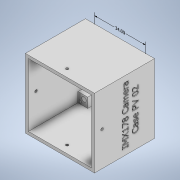
# Autodesk Inventor part: IMX178 Camera Case Base
Saved by Autodesk Inventor 2022.1 (Build 261234000, 234)
## iProperties
Created: 2021-07-23
Part Number: IMX178 Camera Case Base
Material: Generic
Document SubType Name: Modeling
Designer: robst
Density: 1 g/cm^3
Appearance: Default
Author: robst
Autodesk Inventor part; units mm, degrees
ref_plane "YZ Plane" through (0, 0, 0) normal (1, 0, 0) x (0, 1, 0)
ref_plane "XZ Plane" through (0, 0, 0) normal (0, 1, 0) x (-1, 0, 0)
ref_plane "XY Plane" through (0, 0, 0) normal (0, 0, 1) x (1, 0, 0)
sketch "Sketch8" plane through (0, 0, 0) normal (0, 0, 1) x (1, 0, 0)
  line L0 (-17, -17) -> (17, -17) construction
  line L1 (17, -17) -> (17, 17) construction
  line L2 (17, 17) -> (-17, 17) construction
  line L3 (-17, 17) -> (-17, -17) construction
  line L4 (-17, -17) -> (17, 17) construction
  line L5 (17, -17) -> (-17, 17) construction
  circle A0 centre (-17, 17) radius 1.5
  circle A1 centre (17, 17) radius 1.5
  circle A2 centre (17, -17) radius 1.5
  circle A3 centre (-17, -17) radius 1.5
  line L6 (-21, -21) -> (21, -21)
  line L7 (21, -21) -> (21, 21)
  line L8 (21, 21) -> (-21, 21)
  line L9 (-21, 21) -> (-21, -21)
  line L10 (-21, -21) -> (21, 21) construction
  line L11 (21, -21) -> (-21, 21) construction
  line L12 (-23, -23) -> (23, -23)
  line L13 (23, -23) -> (23, 23)
  line L14 (23, 23) -> (-23, 23)
  line L15 (-23, 23) -> (-23, -23)
  line L16 (-23, -23) -> (23, 23) construction
  line L17 (23, -23) -> (-23, 23) construction
  line L18 (0, 0) -> (9.8286, 0)
  line L19 (-14.5, -14.5) -> (14.5, -14.5) construction
  line L20 (14.5, -14.5) -> (14.5, 14.5) construction
  line L21 (14.5, 14.5) -> (-14.5, 14.5) construction
  line L22 (-14.5, 14.5) -> (-14.5, -14.5) construction
  line L23 (-14.5, -14.5) -> (14.5, 14.5) construction
  line L24 (14.5, -14.5) -> (-14.5, 14.5) construction
  line L25 (-21, 21) -> (-14.5, 21)
  line L26 (-14.5, 21) -> (-14.5, 14.5)
  line L27 (-14.5, 14.5) -> (-21, 14.5)
  line L28 (-21, 14.5) -> (-21, 21)
  line L29 (21, 21) -> (14.5, 21)
  line L30 (14.5, 21) -> (14.5, 14.5)
  line L31 (14.5, 14.5) -> (21, 14.5)
  line L32 (21, 14.5) -> (21, 21)
  line L33 (21, -21) -> (14.5, -21)
  line L34 (14.5, -21) -> (14.5, -14.5)
  line L35 (14.5, -14.5) -> (21, -14.5)
  line L36 (21, -14.5) -> (21, -21)
  line L37 (-21, -21) -> (-14.5, -21)
  line L38 (-14.5, -21) -> (-14.5, -14.5)
  line L39 (-14.5, -14.5) -> (-21, -14.5)
  line L40 (-21, -14.5) -> (-21, -21)
  point P0 (-23, 0)
  dimension "d46" = 34
  dimension "d47" = 34
  dimension "d48" = 3
  dimension "d49" = 42
  dimension "d50" = 42
  dimension "d51" = 2
  dimension "d52" = 2
  dimension "d53" = 29
  dimension "d54" = 29
  constraints: 82 end point, 16 parallel, 9 midpoint, 8 horizontal, 8 perpendicular, 4 centre point, 4 coincident, 3 equal radius, 2 point on line
  measures "d46" distance of L0.start L0.end
  measures "d47" distance of L2.end L0.start
  measures "d48" diameter of A0
  measures "d49" distance of L7.end L8.end
  measures "d50" distance of L6.end L7.end
  measures "d51" distance between parallel lines of L8 L14
  measures "d52" distance from line of point (-23, 0) L9
  measures "d53" distance of L19.start L19.end
  measures "d54" distance of L20.end L19.end
extrude "Extrusion9" add sketch "Sketch8" against normal blind 15 contours L9 L39 L38 L6 | L34 L35 L7 L6 | L9 L8 L26 L27 | L31 L30 L8 L7 | L15 L14 L13 L12
sketch "Sketch9" plane through (0, 0, 0) normal (0, 0, 1) x (1, 0, 0)
  line L0 (21, 14.5) -> (21, -14.5) projected
  line L1 (-14.5, 21) -> (14.5, 21) projected
  line L2 (-21, -14.5) -> (-21, 14.5) projected
  line L3 (14.5, -21) -> (-14.5, -21) projected
  line L4 (-23, -23) -> (23, -23) projected
  line L5 (23, -23) -> (23, 23) projected
  line L6 (23, 23) -> (-23, 23) projected
  line L7 (-23, 23) -> (-23, -23) projected
  line L8 (-21, -21) -> (21, -21)
  line L9 (21, -21) -> (21, 21)
  line L10 (21, 21) -> (-21, 21)
  line L11 (-21, 21) -> (-21, -21)
  line L12 (-21, -21) -> (21, 21) construction
  line L13 (21, -21) -> (-21, 21) construction
  line L14 (-23, -23) -> (23, -23)
  line L15 (23, -23) -> (23, 23)
  line L16 (23, 23) -> (-23, 23)
  line L17 (-23, 23) -> (-23, -23)
  line L18 (-23, -23) -> (23, 23) construction
  line L19 (23, -23) -> (-23, 23) construction
  point P0 (0, 0)
  constraints: 24 end point, 4 midpoint, 4 parallel, 2 perpendicular
extrude "Extrusion10" add sketch "Sketch9" along normal blind 25
sketch "Sketch10" plane through (23, -23, -15) normal (1, 0, 0) x (0, 0, -1)
  line L0 (-40, 0) -> (0, 0) construction
  line L1 (-20, 0) -> (-20, 46) construction
  line L2 (0, 46) -> (-40, 46) construction
  line L3 (-17.5, 5.4068) -> (-17.5, 3.8574)
  line L4 (-17.5, 3.8574) -> (-17.9084, 3.8574)
  line L5 (-17.9084, 3.8574) -> (-17.9084, 4.3663)
  line L6 (-17.9084, 4.3663) -> (-21.0916, 4.3663)
  line L7 (-21.0916, 4.3663) -> (-21.0916, 3.8574)
  line L8 (-21.0916, 3.8574) -> (-21.5, 3.8574)
  line L9 (-21.5, 3.8574) -> (-21.5, 5.4068)
  line L10 (-21.5, 5.4068) -> (-21.0916, 5.4068)
  line L11 (-21.0916, 5.4068) -> (-21.0916, 4.8979)
  line L12 (-21.0916, 4.8979) -> (-17.9084, 4.8979)
  line L13 (-17.9084, 4.8979) -> (-17.9084, 5.4068)
  line L14 (-17.9084, 5.4068) -> (-17.5, 5.4068)
  line L15 (-17.5, 9.4943) -> (-17.5, 8.9627)
  line L16 (-17.5, 8.9627) -> (-20.9457, 8.9627)
  line L17 (-20.9457, 8.9627) -> (-18.6021, 7.919)
  line L18 (-18.6021, 7.919) -> (-18.6021, 7.5948)
  line L19 (-18.6021, 7.5948) -> (-20.9457, 6.5608)
  line L20 (-20.9457, 6.5608) -> (-17.5, 6.5608)
  line L21 (-17.5, 6.5608) -> (-17.5, 6.0648)
  line L22 (-17.5, 6.0648) -> (-21.5, 6.0648)
  line L23 (-21.5, 6.0648) -> (-21.5, 6.7909)
  line L24 (-21.5, 6.7909) -> (-19.2731, 7.7893)
  line L25 (-19.2731, 7.7893) -> (-21.5, 8.7553)
  line L26 (-21.5, 8.7553) -> (-21.5, 9.4943)
  line L27 (-21.5, 9.4943) -> (-17.5, 9.4943)
  line L28 (-17.5, 13.0697) -> (-17.5, 12.4603)
  line L29 (-17.5, 12.4603) -> (-19.0948, 11.4878)
  line L30 (-19.0948, 11.4878) -> (-17.5, 10.4959)
  line L31 (-17.5, 10.4959) -> (-17.5, 9.9222)
  line L32 (-17.5, 9.9222) -> (-19.5032, 11.1961)
  line L33 (-19.5032, 11.1961) -> (-21.5, 9.9611)
  line L34 (-21.5, 9.9611) -> (-21.5, 10.5705)
  line L35 (-21.5, 10.5705) -> (-19.9344, 11.5235)
  line L36 (-19.9344, 11.5235) -> (-21.5, 12.4959)
  line L37 (-21.5, 12.4959) -> (-21.5, 13.0697)
  line L38 (-21.5, 13.0697) -> (-19.5292, 11.8185)
  line L39 (-19.5292, 11.8185) -> (-17.5, 13.0697)
  line L40 (-17.5, 15.6499) -> (-17.5, 13.6985)
  line L41 (-17.5, 13.6985) -> (-17.9084, 13.6985)
  line L42 (-17.9084, 13.6985) -> (-17.9084, 14.4246)
  line L43 (-17.9084, 14.4246) -> (-20.5891, 14.4246)
  line L44 (-20.5891, 14.4246) -> (-20.5891, 13.6985)
  line L45 (-20.5891, 13.6985) -> (-20.9554, 13.6985)
  spline S0 degree 2 poles (-20.9554, 13.6985) (-20.9554, 14.1102) (-21.1888, 14.4992) (-21.513, 14.5251) knots 0 0 0 1 2 2 2
  line L46 (-21.513, 14.5251) -> (-21.513, 14.94)
  line L47 (-21.513, 14.94) -> (-17.9084, 14.94)
  line L48 (-17.9084, 14.94) -> (-17.9084, 15.6499)
  line L49 (-17.9084, 15.6499) -> (-17.5, 15.6499)
  line L50 (-20.9003, 18.8979) -> (-17.5, 17.1669)
  line L51 (-17.5, 17.1669) -> (-17.5, 16.5964)
  line L52 (-17.5, 16.5964) -> (-21.03, 18.4246)
  line L53 (-21.03, 18.4246) -> (-21.03, 16.3598)
  line L54 (-21.03, 16.3598) -> (-21.5, 16.3598)
  line L55 (-21.5, 16.3598) -> (-21.5, 18.8979)
  line L56 (-21.5, 18.8979) -> (-20.9003, 18.8979)
  spline S1 degree 2 poles (-17.4092, 20.5964) (-17.4092, 20.2982) (-17.5875, 19.8088) (-17.7528, 19.637) knots 0 0 0 1 2 2 2
  spline S2 degree 2 poles (-17.7528, 19.637) (-17.9149, 19.4684) (-18.3558, 19.2934) (-18.6053, 19.2934) knots 0 0 0 1 2 2 2
  spline S3 degree 2 poles (-18.6053, 19.2934) (-18.9295, 19.2934) (-19.4741, 19.6402) (-19.6361, 19.9708) knots 0 0 0 1 2 2 2
  line L57 (-19.6361, 19.9708) -> (-19.6524, 19.9708)
  spline S4 degree 2 poles (-19.6524, 19.9708) (-19.8241, 19.6759) (-20.2326, 19.3906) (-20.5373, 19.3906) knots 0 0 0 1 2 2 2
  spline S5 degree 2 poles (-20.5373, 19.3906) (-20.9878, 19.3906) (-21.5908, 20.0713) (-21.5908, 20.5964) knots 0 0 0 1 2 2 2
  spline S6 degree 2 poles (-21.5908, 20.5964) (-21.5908, 21.141) (-21.0203, 21.799) (-20.5729, 21.799) knots 0 0 0 1 2 2 2
  spline S7 degree 2 poles (-20.5729, 21.799) (-20.3039, 21.799) (-19.7788, 21.4846) (-19.6297, 21.1896) knots 0 0 0 1 2 2 2
  line L58 (-19.6297, 21.1896) -> (-19.6135, 21.1896)
  spline S8 degree 2 poles (-19.6135, 21.1896) (-19.4514, 21.5397) (-18.9846, 21.8995) (-18.6151, 21.8995) knots 0 0 0 1 2 2 2
  spline S9 degree 2 poles (-18.6151, 21.8995) (-18.1029, 21.8995) (-17.4092, 21.154) (-17.4092, 20.5964) knots 0 0 0 1 2 2 2
  spline S10 degree 2 poles (-18.5632, 21.3485) (-18.8096, 21.3485) (-19.1013, 21.154) (-19.2504, 20.8784) knots 0 0 0 1 2 2 2
  spline S11 degree 2 poles (-19.2504, 20.8784) (-19.3023, 20.7877) (-19.4222, 20.483) (-19.5, 20.2917) knots 0 0 0 1 2 2 2
  spline S12 degree 2 poles (-19.5, 20.2917) (-19.3541, 20.0713) (-18.9198, 19.8347) (-18.6442, 19.8347) knots 0 0 0 1 2 2 2
  spline S13 degree 2 poles (-18.6442, 19.8347) (-18.2812, 19.8347) (-17.8079, 20.2723) (-17.8079, 20.6029) knots 0 0 0 1 2 2 2
  spline S14 degree 2 poles (-17.8079, 20.6029) (-17.8079, 20.94) (-18.2131, 21.3485) (-18.5632, 21.3485) knots 0 0 0 1 2 2 2
  spline S15 degree 2 poles (-20.5665, 21.2739) (-20.8355, 21.2739) (-21.1953, 20.9141) (-21.1953, 20.5932) knots 0 0 0 1 2 2 2
  spline S16 degree 2 poles (-21.1953, 20.5932) (-21.1953, 20.3015) (-20.8744, 19.9287) (-20.5989, 19.9287) knots 0 0 0 1 2 2 2
  spline S17 degree 2 poles (-20.5989, 19.9287) (-20.4011, 19.9287) (-20.1256, 20.1199) (-20.0154, 20.3112) knots 0 0 0 1 2 2 2
  spline S18 degree 2 poles (-20.0154, 20.3112) (-19.97, 20.3922) (-19.8112, 20.7358) (-19.7658, 20.8752) knots 0 0 0 1 2 2 2
  spline S19 degree 2 poles (-19.7658, 20.8752) (-19.9441, 21.1086) (-20.3233, 21.2739) (-20.5665, 21.2739) knots 0 0 0 1 2 2 2
  spline S20 degree 2 poles (-17.4287, 25.7828) (-17.4287, 25.3938) (-17.6912, 24.7358) (-17.9538, 24.4959) knots 0 0 0 1 2 2 2
  spline S21 degree 2 poles (-17.9538, 24.4959) (-18.2131, 24.2561) (-18.9911, 23.9935) (-19.4968, 23.9935) knots 0 0 0 1 2 2 2
  spline S22 degree 2 poles (-19.4968, 23.9935) (-19.9992, 23.9935) (-20.7447, 24.2496) (-21.0203, 24.4927) knots 0 0 0 1 2 2 2
  spline S23 degree 2 poles (-21.0203, 24.4927) (-21.2893, 24.7326) (-21.5713, 25.3874) (-21.5713, 25.7925) knots 0 0 0 1 2 2 2
  spline S24 degree 2 poles (-21.5713, 25.7925) (-21.5713, 25.9935) (-21.513, 26.3468) (-21.4676, 26.4959) knots 0 0 0 1 2 2 2
  spline S25 degree 2 poles (-21.4676, 26.4959) (-21.4254, 26.6256) (-21.3055, 26.8947) (-21.2342, 27.0276) knots 0 0 0 1 2 2 2
  line L59 (-21.2342, 27.0276) -> (-20.5924, 27.0276)
  line L60 (-20.5924, 27.0276) -> (-20.5924, 26.9854)
  spline S26 degree 2 poles (-20.5924, 26.9854) (-20.6572, 26.9141) (-20.8387, 26.6937) (-20.9263, 26.5348) knots 0 0 0 1 2 2 2
  spline S27 degree 2 poles (-20.9263, 26.5348) (-21.0105, 26.3825) (-21.1175, 26.0227) (-21.1175, 25.7893) knots 0 0 0 1 2 2 2
  spline S28 degree 2 poles (-21.1175, 25.7893) (-21.1175, 25.5332) (-20.9068, 25.0762) (-20.7058, 24.9044) knots 0 0 0 1 2 2 2
  spline S29 degree 2 poles (-20.7058, 24.9044) (-20.5016, 24.7358) (-19.8825, 24.5478) (-19.4968, 24.5478) knots 0 0 0 1 2 2 2
  spline S30 degree 2 poles (-19.4968, 24.5478) (-19.0851, 24.5478) (-18.4919, 24.7455) (-18.2877, 24.9173) knots 0 0 0 1 2 2 2
  spline S31 degree 2 poles (-18.2877, 24.9173) (-18.09, 25.0859) (-17.889, 25.5365) (-17.889, 25.7893) knots 0 0 0 1 2 2 2
  spline S32 degree 2 poles (-17.889, 25.7893) (-17.889, 26.0194) (-18.0024, 26.4117) (-18.0867, 26.564) knots 0 0 0 1 2 2 2
  spline S33 degree 2 poles (-18.0867, 26.564) (-18.171, 26.7099) (-18.346, 26.9271) (-18.4076, 26.9887) knots 0 0 0 1 2 2 2
  line L61 (-18.4076, 26.9887) -> (-18.4076, 27.0276)
  line L62 (-18.4076, 27.0276) -> (-17.7723, 27.0276)
  spline S34 degree 2 poles (-17.7723, 27.0276) (-17.7107, 26.8947) (-17.5972, 26.6613) (-17.5454, 26.4959) knots 0 0 0 1 2 2 2
  spline S35 degree 2 poles (-17.5454, 26.4959) (-17.487, 26.3209) (-17.4287, 26.0227) (-17.4287, 25.7828) knots 0 0 0 1 2 2 2
  spline S36 degree 2 poles (-17.8177, 29.1572) (-17.7723, 29.0956) (-17.6102, 28.8882) (-17.5616, 28.7909) knots 0 0 0 1 2 2 2
  spline S37 degree 2 poles (-17.5616, 28.7909) (-17.4903, 28.658) (-17.4157, 28.4084) (-17.4157, 28.1815) knots 0 0 0 1 2 2 2
  spline S38 degree 2 poles (-17.4157, 28.1815) (-17.4157, 27.9968) (-17.5551, 27.6629) (-17.6815, 27.5365) knots 0 0 0 1 2 2 2
  spline S39 degree 2 poles (-17.6815, 27.5365) (-17.8047, 27.4165) (-18.1677, 27.2707) (-18.3687, 27.2707) knots 0 0 0 1 2 2 2
  spline S40 degree 2 poles (-18.3687, 27.2707) (-18.6799, 27.2707) (-19.1207, 27.5332) (-19.2472, 27.8185) knots 0 0 0 1 2 2 2
  spline S41 degree 2 poles (-19.2472, 27.8185) (-19.3639, 28.0713) (-19.4514, 28.7585) (-19.4741, 29.1572) knots 0 0 0 1 2 2 2
  line L63 (-19.4741, 29.1572) -> (-19.5713, 29.1572)
  spline S42 degree 2 poles (-19.5713, 29.1572) (-19.7464, 29.1572) (-19.9635, 29.0502) (-20.0251, 28.953) knots 0 0 0 1 2 2 2
  spline S43 degree 2 poles (-20.0251, 28.953) (-20.0867, 28.8558) (-20.1256, 28.577) (-20.1256, 28.4279) knots 0 0 0 1 2 2 2
  spline S44 degree 2 poles (-20.1256, 28.4279) (-20.1256, 28.2528) (-20.0219, 27.7796) (-19.9214, 27.543) knots 0 0 0 1 2 2 2
  line L64 (-19.9214, 27.543) -> (-19.9214, 27.5138)
  line L65 (-19.9214, 27.5138) -> (-20.4368, 27.5138)
  spline S45 degree 2 poles (-20.4368, 27.5138) (-20.4757, 27.6532) (-20.5729, 28.175) (-20.5729, 28.4311) knots 0 0 0 1 2 2 2
  spline S46 degree 2 poles (-20.5729, 28.4311) (-20.5729, 28.7423) (-20.4757, 29.1669) (-20.3493, 29.3355) knots 0 0 0 1 2 2 2
  spline S47 degree 2 poles (-20.3493, 29.3355) (-20.2261, 29.5008) (-19.8339, 29.6629) (-19.5519, 29.6629) knots 0 0 0 1 2 2 2
  line L66 (-19.5519, 29.6629) -> (-17.5, 29.6629)
  line L67 (-17.5, 29.6629) -> (-17.5, 29.1572)
  line L68 (-17.5, 29.1572) -> (-17.8177, 29.1572)
  line L69 (-18.2391, 29.1572) -> (-19.0721, 29.1572)
  spline S48 degree 2 poles (-19.0721, 29.1572) (-19.0559, 28.9757) (-19.0008, 28.4279) (-18.9489, 28.2561) knots 0 0 0 1 2 2 2
  spline S49 degree 2 poles (-18.9489, 28.2561) (-18.8874, 28.0551) (-18.6313, 27.7925) (-18.4044, 27.7925) knots 0 0 0 1 2 2 2
  spline S50 degree 2 poles (-18.4044, 27.7925) (-18.1451, 27.7925) (-17.8825, 28.0843) (-17.8825, 28.363) knots 0 0 0 1 2 2 2
  spline S51 degree 2 poles (-17.8825, 28.363) (-17.8825, 28.5997) (-18.0867, 28.9887) (-18.2391, 29.1572) knots 0 0 0 1 2 2 2
  line L70 (-17.5, 33.7763) -> (-19.2374, 33.7763)
  spline S52 degree 2 poles (-19.2374, 33.7763) (-19.4449, 33.7763) (-19.7982, 33.7439) (-19.8955, 33.6921) knots 0 0 0 1 2 2 2
  spline S53 degree 2 poles (-19.8955, 33.6921) (-20.0024, 33.6402) (-20.1062, 33.4425) (-20.1062, 33.2707) knots 0 0 0 1 2 2 2
  spline S54 degree 2 poles (-20.1062, 33.2707) (-20.1062, 33.1151) (-19.9149, 32.7585) (-19.7334, 32.5705) knots 0 0 0 1 2 2 2
  spline S55 degree 2 poles (-19.7334, 32.5705) (-19.688, 32.5737) (-19.5616, 32.5802) (-19.4773, 32.5802) knots 0 0 0 1 2 2 2
  line L71 (-19.4773, 32.5802) -> (-17.5, 32.5802)
  line L72 (-17.5, 32.5802) -> (-17.5, 32.0746)
  line L73 (-17.5, 32.0746) -> (-19.2374, 32.0746)
  spline S56 degree 2 poles (-19.2374, 32.0746) (-19.4449, 32.0746) (-19.7982, 32.0421) (-19.8955, 31.9903) knots 0 0 0 1 2 2 2
  spline S57 degree 2 poles (-19.8955, 31.9903) (-20.0024, 31.9384) (-20.1062, 31.7407) (-20.1062, 31.5689) knots 0 0 0 1 2 2 2
  spline S58 degree 2 poles (-20.1062, 31.5689) (-20.1062, 31.4068) (-19.9019, 31.047) (-19.7431, 30.8784) knots 0 0 0 1 2 2 2
  line L74 (-19.7431, 30.8784) -> (-17.5, 30.8784)
  line L75 (-17.5, 30.8784) -> (-17.5, 30.3728)
  line L76 (-17.5, 30.3728) -> (-20.5016, 30.3728)
  line L77 (-20.5016, 30.3728) -> (-20.5016, 30.8784)
  line L78 (-20.5016, 30.8784) -> (-20.171, 30.8784)
  spline S59 degree 2 poles (-20.171, 30.8784) (-20.3687, 31.0762) (-20.5859, 31.4652) (-20.5859, 31.6985) knots 0 0 0 1 2 2 2
  spline S60 degree 2 poles (-20.5859, 31.6985) (-20.5859, 31.9643) (-20.3428, 32.376) (-20.0673, 32.483) knots 0 0 0 1 2 2 2
  spline S61 degree 2 poles (-20.0673, 32.483) (-20.3233, 32.7131) (-20.5859, 33.1475) (-20.5859, 33.4003) knots 0 0 0 1 2 2 2
  spline S62 degree 2 poles (-20.5859, 33.4003) (-20.5859, 33.5948) (-20.466, 33.9125) (-20.3298, 34.0292) knots 0 0 0 1 2 2 2
  spline S63 degree 2 poles (-20.3298, 34.0292) (-20.1937, 34.1491) (-19.7853, 34.282) (-19.4773, 34.282) knots 0 0 0 1 2 2 2
  line L79 (-19.4773, 34.282) -> (-17.5, 34.282)
  line L80 (-17.5, 34.282) -> (-17.5, 33.7763)
  spline S64 degree 2 poles (-17.4319, 36.295) (-17.4319, 35.5754) (-18.2391, 34.7844) (-18.9846, 34.7844) knots 0 0 0 1 2 2 2
  spline S65 degree 2 poles (-18.9846, 34.7844) (-19.7172, 34.7844) (-20.5859, 35.5527) (-20.5859, 36.1718) knots 0 0 0 1 2 2 2
  spline S66 degree 2 poles (-20.5859, 36.1718) (-20.5859, 36.4506) (-20.4238, 36.8817) (-20.252, 37.0405) knots 0 0 0 1 2 2 2
  spline S67 degree 2 poles (-20.252, 37.0405) (-20.0802, 37.2026) (-19.5843, 37.3744) (-19.2245, 37.3744) knots 0 0 0 1 2 2 2
  line L81 (-19.2245, 37.3744) -> (-18.9489, 37.3744)
  line L82 (-18.9489, 37.3744) -> (-18.9489, 35.2966)
  spline S68 degree 2 poles (-18.9489, 35.2966) (-18.4271, 35.2966) (-17.8728, 35.8217) (-17.8728, 36.2885) knots 0 0 0 1 2 2 2
  spline S69 degree 2 poles (-17.8728, 36.2885) (-17.8728, 36.4538) (-17.9473, 36.7747) (-18.0057, 36.9044) knots 0 0 0 1 2 2 2
  spline S70 degree 2 poles (-18.0057, 36.9044) (-18.0705, 37.0405) (-18.184, 37.2285) (-18.2358, 37.2901) knots 0 0 0 1 2 2 2
  line L83 (-18.2358, 37.2901) -> (-18.2358, 37.3193)
  line L84 (-18.2358, 37.3193) -> (-17.6848, 37.3193)
  spline S71 degree 2 poles (-17.6848, 37.3193) (-17.6491, 37.2318) (-17.5454, 36.966) (-17.5162, 36.8622) knots 0 0 0 1 2 2 2
  spline S72 degree 2 poles (-17.5162, 36.8622) (-17.4741, 36.7164) (-17.4319, 36.4765) (-17.4319, 36.295) knots 0 0 0 1 2 2 2
  spline S73 degree 2 poles (-19.3347, 36.8817) (-19.5389, 36.8752) (-19.8371, 36.7909) (-19.9376, 36.7099) knots 0 0 0 1 2 2 2
  spline S74 degree 2 poles (-19.9376, 36.7099) (-20.0511, 36.6224) (-20.171, 36.3468) (-20.171, 36.1426) knots 0 0 0 1 2 2 2
  spline S75 degree 2 poles (-20.171, 36.1426) (-20.171, 35.9417) (-20.0511, 35.6596) (-19.9344, 35.543) knots 0 0 0 1 2 2 2
  spline S76 degree 2 poles (-19.9344, 35.543) (-19.8144, 35.4295) (-19.5259, 35.3128) (-19.3347, 35.2966) knots 0 0 0 1 2 2 2
  line L85 (-19.3347, 35.2966) -> (-19.3347, 36.8817)
  line L86 (-19.9603, 39.4781) -> (-19.9603, 39.4522)
  spline S77 degree 2 poles (-19.9603, 39.4522) (-19.9765, 39.3938) (-19.983, 39.2674) (-19.983, 39.1799) knots 0 0 0 1 2 2 2
  spline S78 degree 2 poles (-19.983, 39.1799) (-19.983, 38.9757) (-19.8047, 38.5737) (-19.6297, 38.3922) knots 0 0 0 1 2 2 2
  line L87 (-19.6297, 38.3922) -> (-17.5, 38.3922)
  line L88 (-17.5, 38.3922) -> (-17.5, 37.8865)
  line L89 (-17.5, 37.8865) -> (-20.5016, 37.8865)
  line L90 (-20.5016, 37.8865) -> (-20.5016, 38.3922)
  line L91 (-20.5016, 38.3922) -> (-20.0543, 38.3922)
  spline S79 degree 2 poles (-20.0543, 38.3922) (-20.3006, 38.6677) (-20.5016, 39.0794) (-20.5016, 39.2739) knots 0 0 0 1 2 2 2
  spline S80 degree 2 poles (-20.5016, 39.2739) (-20.5016, 39.3517) (-20.4951, 39.4295) (-20.4854, 39.4781) knots 0 0 0 1 2 2 2
  line L92 (-20.4854, 39.4781) -> (-19.9603, 39.4781)
  spline S81 degree 2 poles (-17.8177, 41.543) (-17.7723, 41.4814) (-17.6102, 41.2739) (-17.5616, 41.1767) knots 0 0 0 1 2 2 2
  spline S82 degree 2 poles (-17.5616, 41.1767) (-17.4903, 41.0438) (-17.4157, 40.7942) (-17.4157, 40.5673) knots 0 0 0 1 2 2 2
  spline S83 degree 2 poles (-17.4157, 40.5673) (-17.4157, 40.3825) (-17.5551, 40.0486) (-17.6815, 39.9222) knots 0 0 0 1 2 2 2
  spline S84 degree 2 poles (-17.6815, 39.9222) (-17.8047, 39.8023) (-18.1677, 39.6564) (-18.3687, 39.6564) knots 0 0 0 1 2 2 2
  spline S85 degree 2 poles (-18.3687, 39.6564) (-18.6799, 39.6564) (-19.1207, 39.919) (-19.2472, 40.2042) knots 0 0 0 1 2 2 2
  spline S86 degree 2 poles (-19.2472, 40.2042) (-19.3639, 40.4571) (-19.4514, 41.1442) (-19.4741, 41.543) knots 0 0 0 1 2 2 2
  line L93 (-19.4741, 41.543) -> (-19.5713, 41.543)
  spline S87 degree 2 poles (-19.5713, 41.543) (-19.7464, 41.543) (-19.9635, 41.436) (-20.0251, 41.3387) knots 0 0 0 1 2 2 2
  spline S88 degree 2 poles (-20.0251, 41.3387) (-20.0867, 41.2415) (-20.1256, 40.9627) (-20.1256, 40.8136) knots 0 0 0 1 2 2 2
  spline S89 degree 2 poles (-20.1256, 40.8136) (-20.1256, 40.6386) (-20.0219, 40.1653) (-19.9214, 39.9287) knots 0 0 0 1 2 2 2
  line L94 (-19.9214, 39.9287) -> (-19.9214, 39.8995)
  line L95 (-19.9214, 39.8995) -> (-20.4368, 39.8995)
  spline S90 degree 2 poles (-20.4368, 39.8995) (-20.4757, 40.0389) (-20.5729, 40.5608) (-20.5729, 40.8169) knots 0 0 0 1 2 2 2
  spline S91 degree 2 poles (-20.5729, 40.8169) (-20.5729, 41.128) (-20.4757, 41.5527) (-20.3493, 41.7212) knots 0 0 0 1 2 2 2
  spline S92 degree 2 poles (-20.3493, 41.7212) (-20.2261, 41.8865) (-19.8339, 42.0486) (-19.5519, 42.0486) knots 0 0 0 1 2 2 2
  line L96 (-19.5519, 42.0486) -> (-17.5, 42.0486)
  line L97 (-17.5, 42.0486) -> (-17.5, 41.543)
  line L98 (-17.5, 41.543) -> (-17.8177, 41.543)
  line L99 (-18.2391, 41.543) -> (-19.0721, 41.543)
  spline S93 degree 2 poles (-19.0721, 41.543) (-19.0559, 41.3614) (-19.0008, 40.8136) (-18.9489, 40.6418) knots 0 0 0 1 2 2 2
  spline S94 degree 2 poles (-18.9489, 40.6418) (-18.8874, 40.4408) (-18.6313, 40.1783) (-18.4044, 40.1783) knots 0 0 0 1 2 2 2
  spline S95 degree 2 poles (-18.4044, 40.1783) (-18.1451, 40.1783) (-17.8825, 40.47) (-17.8825, 40.7488) knots 0 0 0 1 2 2 2
  spline S96 degree 2 poles (-17.8825, 40.7488) (-17.8825, 40.9854) (-18.0867, 41.3744) (-18.2391, 41.543) knots 0 0 0 1 2 2 2
  spline S97 degree 2 poles (-10.8233, 11.3193) (-10.8233, 10.9303) (-11.0858, 10.2723) (-11.3484, 10.0324) knots 0 0 0 1 2 2 2
  spline S98 degree 2 poles (-11.3484, 10.0324) (-11.6077, 9.7925) (-12.3856, 9.53) (-12.8913, 9.53) knots 0 0 0 1 2 2 2
  spline S99 degree 2 poles (-12.8913, 9.53) (-13.3938, 9.53) (-14.1393, 9.7861) (-14.4148, 10.0292) knots 0 0 0 1 2 2 2
  spline S100 degree 2 poles (-14.4148, 10.0292) (-14.6839, 10.269) (-14.9659, 10.9238) (-14.9659, 11.329) knots 0 0 0 1 2 2 2
  spline S101 degree 2 poles (-14.9659, 11.329) (-14.9659, 11.53) (-14.9075, 11.8833) (-14.8621, 12.0324) knots 0 0 0 1 2 2 2
  spline S102 degree 2 poles (-14.8621, 12.0324) (-14.82, 12.1621) (-14.7001, 12.4311) (-14.6288, 12.564) knots 0 0 0 1 2 2 2
  line L100 (-14.6288, 12.564) -> (-13.9869, 12.564)
  line L101 (-13.9869, 12.564) -> (-13.9869, 12.5219)
  spline S103 degree 2 poles (-13.9869, 12.5219) (-14.0518, 12.4506) (-14.2333, 12.2301) (-14.3208, 12.0713) knots 0 0 0 1 2 2 2
  spline S104 degree 2 poles (-14.3208, 12.0713) (-14.4051, 11.919) (-14.5121, 11.5592) (-14.5121, 11.3258) knots 0 0 0 1 2 2 2
  spline S105 degree 2 poles (-14.5121, 11.3258) (-14.5121, 11.0697) (-14.3014, 10.6126) (-14.1004, 10.4408) knots 0 0 0 1 2 2 2
  spline S106 degree 2 poles (-14.1004, 10.4408) (-13.8962, 10.2723) (-13.2771, 10.0843) (-12.8913, 10.0843) knots 0 0 0 1 2 2 2
  spline S107 degree 2 poles (-12.8913, 10.0843) (-12.4797, 10.0843) (-11.8865, 10.282) (-11.6822, 10.4538) knots 0 0 0 1 2 2 2
  spline S108 degree 2 poles (-11.6822, 10.4538) (-11.4845, 10.6224) (-11.2835, 11.0729) (-11.2835, 11.3258) knots 0 0 0 1 2 2 2
  spline S109 degree 2 poles (-11.2835, 11.3258) (-11.2835, 11.5559) (-11.397, 11.9481) (-11.4813, 12.1005) knots 0 0 0 1 2 2 2
  spline S110 degree 2 poles (-11.4813, 12.1005) (-11.5656, 12.2464) (-11.7406, 12.4635) (-11.8022, 12.5251) knots 0 0 0 1 2 2 2
  line L102 (-11.8022, 12.5251) -> (-11.8022, 12.564)
  line L103 (-11.8022, 12.564) -> (-11.1668, 12.564)
  spline S111 degree 2 poles (-11.1668, 12.564) (-11.1053, 12.4311) (-10.9918, 12.1977) (-10.9399, 12.0324) knots 0 0 0 1 2 2 2
  spline S112 degree 2 poles (-10.9399, 12.0324) (-10.8816, 11.8574) (-10.8233, 11.5592) (-10.8233, 11.3193) knots 0 0 0 1 2 2 2
  spline S113 degree 2 poles (-11.2122, 14.6937) (-11.1668, 14.6321) (-11.0048, 14.4246) (-10.9562, 14.3274) knots 0 0 0 1 2 2 2
  spline S114 degree 2 poles (-10.9562, 14.3274) (-10.8848, 14.1945) (-10.8103, 13.9449) (-10.8103, 13.718) knots 0 0 0 1 2 2 2
  spline S115 degree 2 poles (-10.8103, 13.718) (-10.8103, 13.5332) (-10.9497, 13.1994) (-11.0761, 13.0729) knots 0 0 0 1 2 2 2
  spline S116 degree 2 poles (-11.0761, 13.0729) (-11.1993, 12.953) (-11.5623, 12.8071) (-11.7633, 12.8071) knots 0 0 0 1 2 2 2
  spline S117 degree 2 poles (-11.7633, 12.8071) (-12.0745, 12.8071) (-12.5153, 13.0697) (-12.6417, 13.3549) knots 0 0 0 1 2 2 2
  spline S118 degree 2 poles (-12.6417, 13.3549) (-12.7584, 13.6078) (-12.8459, 14.295) (-12.8686, 14.6937) knots 0 0 0 1 2 2 2
  line L104 (-12.8686, 14.6937) -> (-12.9659, 14.6937)
  spline S119 degree 2 poles (-12.9659, 14.6937) (-13.1409, 14.6937) (-13.3581, 14.5867) (-13.4197, 14.4895) knots 0 0 0 1 2 2 2
  spline S120 degree 2 poles (-13.4197, 14.4895) (-13.4813, 14.3922) (-13.5202, 14.1135) (-13.5202, 13.9643) knots 0 0 0 1 2 2 2
  spline S121 degree 2 poles (-13.5202, 13.9643) (-13.5202, 13.7893) (-13.4164, 13.316) (-13.316, 13.0794) knots 0 0 0 1 2 2 2
  line L105 (-13.316, 13.0794) -> (-13.316, 13.0502)
  line L106 (-13.316, 13.0502) -> (-13.8314, 13.0502)
  spline S122 degree 2 poles (-13.8314, 13.0502) (-13.8703, 13.1896) (-13.9675, 13.7115) (-13.9675, 13.9676) knots 0 0 0 1 2 2 2
  spline S123 degree 2 poles (-13.9675, 13.9676) (-13.9675, 14.2788) (-13.8703, 14.7034) (-13.7438, 14.872) knots 0 0 0 1 2 2 2
  spline S124 degree 2 poles (-13.7438, 14.872) (-13.6207, 15.0373) (-13.2284, 15.1994) (-12.9464, 15.1994) knots 0 0 0 1 2 2 2
  line L107 (-12.9464, 15.1994) -> (-10.8946, 15.1994)
  line L108 (-10.8946, 15.1994) -> (-10.8946, 14.6937)
  line L109 (-10.8946, 14.6937) -> (-11.2122, 14.6937)
  line L110 (-11.6336, 14.6937) -> (-12.4667, 14.6937)
  spline S125 degree 2 poles (-12.4667, 14.6937) (-12.4505, 14.5122) (-12.3954, 13.9643) (-12.3435, 13.7925) knots 0 0 0 1 2 2 2
  spline S126 degree 2 poles (-12.3435, 13.7925) (-12.2819, 13.5916) (-12.0258, 13.329) (-11.7989, 13.329) knots 0 0 0 1 2 2 2
  spline S127 degree 2 poles (-11.7989, 13.329) (-11.5396, 13.329) (-11.2771, 13.6207) (-11.2771, 13.8995) knots 0 0 0 1 2 2 2
  spline S128 degree 2 poles (-11.2771, 13.8995) (-11.2771, 14.1361) (-11.4813, 14.5251) (-11.6336, 14.6937) knots 0 0 0 1 2 2 2
  spline S129 degree 2 poles (-10.8233, 16.7196) (-10.8233, 16.4182) (-10.9853, 15.8963) (-11.0761, 15.7245) knots 0 0 0 1 2 2 2
  line L111 (-11.0761, 15.7245) -> (-11.6433, 15.7245)
  line L112 (-11.6433, 15.7245) -> (-11.6433, 15.7504)
  spline S130 degree 2 poles (-11.6433, 15.7504) (-11.5915, 15.8152) (-11.4683, 15.9903) (-11.4002, 16.1361) knots 0 0 0 1 2 2 2
  spline S131 degree 2 poles (-11.4002, 16.1361) (-11.3386, 16.2626) (-11.2479, 16.5737) (-11.2479, 16.7391) knots 0 0 0 1 2 2 2
  spline S132 degree 2 poles (-11.2479, 16.7391) (-11.2479, 16.859) (-11.303, 17.1345) (-11.3484, 17.1994) knots 0 0 0 1 2 2 2
  spline S133 degree 2 poles (-11.3484, 17.1994) (-11.41, 17.2934) (-11.5493, 17.3776) (-11.692, 17.3776) knots 0 0 0 1 2 2 2
  spline S134 degree 2 poles (-11.692, 17.3776) (-11.8703, 17.3776) (-12.055, 17.1831) (-12.1166, 16.9335) knots 0 0 0 1 2 2 2
  spline S135 degree 2 poles (-12.1166, 16.9335) (-12.1393, 16.8363) (-12.2041, 16.5251) (-12.2398, 16.3922) knots 0 0 0 1 2 2 2
  spline S136 degree 2 poles (-12.2398, 16.3922) (-12.3403, 16.0486) (-12.7552, 15.7374) (-13.0502, 15.7374) knots 0 0 0 1 2 2 2
  spline S137 degree 2 poles (-13.0502, 15.7374) (-13.4586, 15.7374) (-13.9675, 16.3501) (-13.9675, 16.8558) knots 0 0 0 1 2 2 2
  spline S138 degree 2 poles (-13.9675, 16.8558) (-13.9675, 17.1053) (-13.8443, 17.611) (-13.7503, 17.7828) knots 0 0 0 1 2 2 2
  line L113 (-13.7503, 17.7828) -> (-13.209, 17.7828)
  line L114 (-13.209, 17.7828) -> (-13.209, 17.7569)
  spline S139 degree 2 poles (-13.209, 17.7569) (-13.3646, 17.5624) (-13.5429, 17.0891) (-13.5429, 16.846) knots 0 0 0 1 2 2 2
  spline S140 degree 2 poles (-13.5429, 16.846) (-13.5429, 16.5964) (-13.3322, 16.2528) (-13.1215, 16.2528) knots 0 0 0 1 2 2 2
  spline S141 degree 2 poles (-13.1215, 16.2528) (-12.9302, 16.2528) (-12.7455, 16.457) (-12.6871, 16.684) knots 0 0 0 1 2 2 2
  spline S142 degree 2 poles (-12.6871, 16.684) (-12.6579, 16.7942) (-12.5996, 17.0729) (-12.5639, 17.2253) knots 0 0 0 1 2 2 2
  spline S143 degree 2 poles (-12.5639, 17.2253) (-12.4797, 17.5559) (-12.0939, 17.893) (-11.76, 17.893) knots 0 0 0 1 2 2 2
  spline S144 degree 2 poles (-11.76, 17.893) (-11.5656, 17.893) (-11.222, 17.7407) (-11.0955, 17.5916) knots 0 0 0 1 2 2 2
  spline S145 degree 2 poles (-11.0955, 17.5916) (-10.9626, 17.4327) (-10.8233, 17.0276) (-10.8233, 16.7196) knots 0 0 0 1 2 2 2
  spline S146 degree 2 poles (-10.8265, 19.6661) (-10.8265, 18.9465) (-11.6336, 18.1556) (-12.3792, 18.1556) knots 0 0 0 1 2 2 2
  spline S147 degree 2 poles (-12.3792, 18.1556) (-13.1117, 18.1556) (-13.9805, 18.9238) (-13.9805, 19.5429) knots 0 0 0 1 2 2 2
  spline S148 degree 2 poles (-13.9805, 19.5429) (-13.9805, 19.8217) (-13.8184, 20.2528) (-13.6466, 20.4117) knots 0 0 0 1 2 2 2
  spline S149 degree 2 poles (-13.6466, 20.4117) (-13.4748, 20.5737) (-12.9788, 20.7455) (-12.619, 20.7455) knots 0 0 0 1 2 2 2
  line L115 (-12.619, 20.7455) -> (-12.3435, 20.7455)
  line L116 (-12.3435, 20.7455) -> (-12.3435, 18.6677)
  spline S150 degree 2 poles (-12.3435, 18.6677) (-11.8216, 18.6677) (-11.2673, 19.1929) (-11.2673, 19.6596) knots 0 0 0 1 2 2 2
  spline S151 degree 2 poles (-11.2673, 19.6596) (-11.2673, 19.825) (-11.3419, 20.1459) (-11.4002, 20.2755) knots 0 0 0 1 2 2 2
  spline S152 degree 2 poles (-11.4002, 20.2755) (-11.4651, 20.4117) (-11.5785, 20.5997) (-11.6304, 20.6613) knots 0 0 0 1 2 2 2
  line L117 (-11.6304, 20.6613) -> (-11.6304, 20.6904)
  line L118 (-11.6304, 20.6904) -> (-11.0793, 20.6904)
  spline S153 degree 2 poles (-11.0793, 20.6904) (-11.0437, 20.6029) (-10.9399, 20.3371) (-10.9108, 20.2334) knots 0 0 0 1 2 2 2
  spline S154 degree 2 poles (-10.9108, 20.2334) (-10.8686, 20.0875) (-10.8265, 19.8476) (-10.8265, 19.6661) knots 0 0 0 1 2 2 2
  spline S155 degree 2 poles (-12.7292, 20.2528) (-12.9335, 20.2464) (-13.2317, 20.1621) (-13.3322, 20.081) knots 0 0 0 1 2 2 2
  spline S156 degree 2 poles (-13.3322, 20.081) (-13.4456, 19.9935) (-13.5656, 19.718) (-13.5656, 19.5138) knots 0 0 0 1 2 2 2
  spline S157 degree 2 poles (-13.5656, 19.5138) (-13.5656, 19.3128) (-13.4456, 19.0308) (-13.3289, 18.9141) knots 0 0 0 1 2 2 2
  spline S158 degree 2 poles (-13.3289, 18.9141) (-13.209, 18.8006) (-12.9205, 18.684) (-12.7292, 18.6677) knots 0 0 0 1 2 2 2
  line L119 (-12.7292, 18.6677) -> (-12.7292, 20.2528)
  spline S159 degree 2 poles (-13.6887, 25.5429) (-13.4294, 25.5429) (-12.9626, 25.3582) (-12.8006, 25.1929) knots 0 0 0 1 2 2 2
  spline S160 degree 2 poles (-12.8006, 25.1929) (-12.5963, 24.9854) (-12.3856, 24.4246) (-12.3856, 23.9968) knots 0 0 0 1 2 2 2
  line L120 (-12.3856, 23.9968) -> (-12.3856, 23.5462)
  line L121 (-12.3856, 23.5462) -> (-10.8946, 23.5462)
  line L122 (-10.8946, 23.5462) -> (-10.8946, 23.0146)
  line L123 (-10.8946, 23.0146) -> (-14.8946, 23.0146)
  line L124 (-14.8946, 23.0146) -> (-14.8946, 24.0194)
  spline S161 degree 2 poles (-14.8946, 24.0194) (-14.8946, 24.376) (-14.7779, 24.8752) (-14.645, 25.0665) knots 0 0 0 1 2 2 2
  spline S162 degree 2 poles (-14.645, 25.0665) (-14.4926, 25.2901) (-14.0226, 25.5429) (-13.6887, 25.5429) knots 0 0 0 1 2 2 2
  spline S163 degree 2 poles (-13.6725, 24.9887) (-13.88, 24.9887) (-14.1847, 24.846) (-14.2819, 24.7002) knots 0 0 0 1 2 2 2
  spline S164 degree 2 poles (-14.2819, 24.7002) (-14.3662, 24.5737) (-14.4343, 24.2366) (-14.4343, 23.987) knots 0 0 0 1 2 2 2
  line L125 (-14.4343, 23.987) -> (-14.4343, 23.5462)
  line L126 (-14.4343, 23.5462) -> (-12.8395, 23.5462)
  line L127 (-12.8395, 23.5462) -> (-12.8395, 23.9092)
  spline S165 degree 2 poles (-12.8395, 23.9092) (-12.8395, 24.2334) (-12.9432, 24.6321) (-13.0793, 24.7618) knots 0 0 0 1 2 2 2
  spline S166 degree 2 poles (-13.0793, 24.7618) (-13.1993, 24.8817) (-13.4813, 24.9887) (-13.6725, 24.9887) knots 0 0 0 1 2 2 2
  line L128 (-14.8946, 28.9498) -> (-10.8946, 27.5721)
  line L129 (-10.8946, 27.5721) -> (-10.8946, 26.9984)
  line L130 (-10.8946, 26.9984) -> (-14.8946, 25.6207)
  line L131 (-14.8946, 25.6207) -> (-14.8946, 26.1912)
  line L132 (-14.8946, 26.1912) -> (-11.572, 27.2998)
  line L133 (-11.572, 27.2998) -> (-14.8946, 28.4084)
  line L134 (-14.8946, 28.4084) -> (-14.8946, 28.9498)
  spline S167 degree 2 poles (-12.8946, 33.4716) (-11.8184, 33.4716) (-10.8103, 32.846) (-10.8103, 32.1945) knots 0 0 0 1 2 2 2
  spline S168 degree 2 poles (-10.8103, 32.1945) (-10.8103, 31.5332) (-11.8378, 30.9141) (-12.8913, 30.9141) knots 0 0 0 1 2 2 2
  spline S169 degree 2 poles (-12.8913, 30.9141) (-13.974, 30.9141) (-14.9756, 31.5397) (-14.9756, 32.1945) knots 0 0 0 1 2 2 2
  spline S170 degree 2 poles (-14.9756, 32.1945) (-14.9756, 32.8525) (-13.9383, 33.4716) (-12.8946, 33.4716) knots 0 0 0 1 2 2 2
  spline S171 degree 2 poles (-11.6758, 32.7844) (-11.8735, 32.8622) (-12.4829, 32.9271) (-12.8946, 32.9271) knots 0 0 0 1 2 2 2
  spline S172 degree 2 poles (-12.8946, 32.9271) (-13.3062, 32.9271) (-13.9124, 32.8622) (-14.1166, 32.7812) knots 0 0 0 1 2 2 2
  spline S173 degree 2 poles (-14.1166, 32.7812) (-14.3208, 32.7002) (-14.5315, 32.4182) (-14.5315, 32.1945) knots 0 0 0 1 2 2 2
  spline S174 degree 2 poles (-14.5315, 32.1945) (-14.5315, 31.9708) (-14.3208, 31.6823) (-14.1101, 31.5981) knots 0 0 0 1 2 2 2
  spline S175 degree 2 poles (-14.1101, 31.5981) (-13.9059, 31.517) (-13.2835, 31.4587) (-12.8913, 31.4587) knots 0 0 0 1 2 2 2
  spline S176 degree 2 poles (-12.8913, 31.4587) (-12.4699, 31.4587) (-11.9059, 31.5105) (-11.6855, 31.5948) knots 0 0 0 1 2 2 2
  spline S177 degree 2 poles (-11.6855, 31.5948) (-11.478, 31.6726) (-11.2544, 31.9611) (-11.2544, 32.1945) knots 0 0 0 1 2 2 2
  spline S178 degree 2 poles (-11.2544, 32.1945) (-11.2544, 32.4149) (-11.4651, 32.7034) (-11.6758, 32.7844) knots 0 0 0 1 2 2 2
  line L135 (-10.8946, 36.4506) -> (-10.8946, 33.9838)
  line L136 (-10.8946, 33.9838) -> (-11.4618, 33.9838)
  spline S179 degree 2 poles (-11.4618, 33.9838) (-11.7114, 34.2496) (-12.175, 34.7229) (-12.4245, 34.9498) knots 0 0 0 1 2 2 2
  spline S180 degree 2 poles (-12.4245, 34.9498) (-12.927, 35.4068) (-13.5299, 35.7407) (-13.8508, 35.7407) knots 0 0 0 1 2 2 2
  spline S181 degree 2 poles (-13.8508, 35.7407) (-14.0194, 35.7407) (-14.2722, 35.637) (-14.3532, 35.5429) knots 0 0 0 1 2 2 2
  spline S182 degree 2 poles (-14.3532, 35.5429) (-14.4343, 35.4489) (-14.5153, 35.2026) (-14.5153, 35.0535) knots 0 0 0 1 2 2 2
  spline S183 degree 2 poles (-14.5153, 35.0535) (-14.5153, 34.9109) (-14.444, 34.6191) (-14.3889, 34.4862) knots 0 0 0 1 2 2 2
  spline S184 degree 2 poles (-14.3889, 34.4862) (-14.3435, 34.3728) (-14.2138, 34.1621) (-14.1685, 34.0972) knots 0 0 0 1 2 2 2
  line L137 (-14.1685, 34.0972) -> (-14.1685, 34.0681)
  line L138 (-14.1685, 34.0681) -> (-14.739, 34.0681)
  spline S185 degree 2 poles (-14.739, 34.0681) (-14.82, 34.2334) (-14.9788, 34.8266) (-14.9788, 35.0924) knots 0 0 0 1 2 2 2
  spline S186 degree 2 poles (-14.9788, 35.0924) (-14.9788, 35.6532) (-14.3856, 36.2853) (-13.88, 36.2853) knots 0 0 0 1 2 2 2
  spline S187 degree 2 poles (-13.88, 36.2853) (-13.6433, 36.2853) (-13.2479, 36.175) (-13.0793, 36.0778) knots 0 0 0 1 2 2 2
  spline S188 degree 2 poles (-13.0793, 36.0778) (-12.9043, 35.9806) (-12.5607, 35.6985) (-12.3954, 35.5429) knots 0 0 0 1 2 2 2
  spline S189 degree 2 poles (-12.3954, 35.5429) (-12.1198, 35.2901) (-11.5299, 34.671) (-11.3581, 34.4862) knots 0 0 0 1 2 2 2
  line L139 (-11.3581, 34.4862) -> (-11.3581, 36.4506)
  line L140 (-11.3581, 36.4506) -> (-10.8946, 36.4506)
  point P0 (-15, 23)
  constraints: 2 end point, 2 midpoint, 1 vertical
emboss "Emboss2" sketch "Sketch10" operation cut depth 1 direction (-1, 0, 0)
sketch "Sketch11" plane through (0, 0, -15) normal (0, 0, -1) x (-1, 0, 0)
  line L0 (-19.5, 19.5) -> (-19.5, -19.5) construction
  line L1 (-19.5, -19.5) -> (19.5, -19.5) construction
  line L2 (19.5, -19.5) -> (19.5, 19.5) construction
  line L3 (19.5, 19.5) -> (-19.5, 19.5) construction
  line L4 (-19.5, 19.5) -> (19.5, -19.5) construction
  line L5 (-19.5, -19.5) -> (19.5, 19.5) construction
  point P0 (0, 0)
  dimension "d61" = 39
  dimension "d62" = 39
  constraints: 12 end point, 4 coincident, 2 midpoint, 2 parallel, 1 perpendicular, 1 vertical
  measures "d61" distance of L0.start L0.end
  measures "d62" distance of L1.end L0.end
hole "Hole1" at (-19.5, 19.5, -15) at (-19.5, -19.5, -15) at (19.5, -19.5, -15) at (19.5, 19.5, -15) direction (0, 0, 1) diameter 1.6942 end through all thread size "2-56 UNC" class "2B" standard "ANSI Unified Screw Threads"
sketch "Sketch12" plane through (-23, -23, -15) normal (-1, 0, 0) x (0, 0, 1)
  line L0 (40, -1) -> (40, 46) projected
  line L1 (30, -3) -> (30, 48) projected
  line L2 (40, 2) -> (40, 44) construction
  line L3 (40, 23) -> (30, 22.5) construction
  point P0 (15, 23)
  point P1 (35, 22.75)
  constraints: 3 midpoint, 2 end point
hole "Hole2" at (-23, -0.25, 20) direction (1, 0, 0) diameter 1.6942 end through all thread size "2-56 UNC" class "2B" standard "ANSI Unified Screw Threads"
sketch "Sketch13" plane through (-23, -23, -15) normal (0, -1, 0) x (1, 0, 0)
  line L0 (0, 40) -> (46, 40) projected
  line L1 (48, 30) -> (-3, 30) projected
  line L2 (2, 40) -> (44, 40) construction
  line L3 (23, 40) -> (22.5, 30) construction
  point P0 (23, 15)
  point P1 (22.75, 35)
  constraints: 3 midpoint, 2 end point
hole "Hole3" at (-0.25, -23, 20) direction (0, 1, 0) diameter 1.6942 end through all thread size "2-56 UNC" class "2B" standard "ANSI Unified Screw Threads"
sketch "Sketch14" plane through (0, 0, 0) normal (0, 0, 1) x (1, 0, 0)
  line L0 (-21, 14.5) -> (-21, -14.5) projected
  line L1 (-21, 21) -> (-21, 14.5) projected
  line L2 (-14.5, 21) -> (-21, 21) projected
  line L3 (14.5, 21) -> (-14.5, 21) projected
  line L4 (21, 21) -> (14.5, 21) projected
  line L5 (21, 14.5) -> (21, 21) projected
  line L6 (21, -14.5) -> (21, 14.5) projected
  line L7 (21, -21) -> (21, -14.5) projected
  line L8 (14.5, -21) -> (21, -21) projected
  line L9 (-14.5, -21) -> (14.5, -21) projected
  line L10 (-21, -21) -> (-14.5, -21) projected
  line L11 (-21, -14.5) -> (-21, -21) projected
  line L12 (-21, -21) -> (21, -21)
  line L13 (21, -21) -> (21, 21)
  line L14 (21, 21) -> (-21, 21)
  line L15 (-21, 21) -> (-21, -21)
  point P0 (0, 0)
  constraints: 8 end point, 2 parallel, 1 horizontal, 1 perpendicular
extrude "Extrusion11" cut sketch "Sketch14" against normal blind 8
equation "\"d46\" = screwSpacing"
equation "\"d47\" = screwSpacing"
equation "\"d48\" = holeDiameter"
equation "\"d49\" = interiorWidth"
equation "\"d50\" = interiorWidth"
equation "\"d51\" = wallThickness"
equation "\"d52\" = wallThickness"
equation "\"screwSpacing\" = 34"
equation "\"interiorWidth\" = 42"
equation "\"wallThickness\" = 2"
equation "\"holeDiameter\" = 3"
body "Solid4"
body "Solid5"
